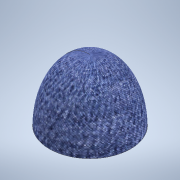
# Autodesk Inventor part: Egg Capsule Top
Saved by Autodesk Inventor 2022 (Build 260153000, 153)
## iProperties
Created: 2022-02-15
Part Number: Egg Capsule Top
Material: Generic
Document SubType Name: Modeling
Designer: Nathan Griffith
Density: 1 g/cm^3
Appearance: Denim - Blue
Author: Nathan Griffith
Autodesk Inventor part; units mm, degrees
ref_plane "YZ Plane" through (0, 0, 0) normal (1, 0, 0) x (0, 1, 0)
ref_plane "XZ Plane" through (0, 0, 0) normal (0, 1, 0) x (-1, 0, 0)
ref_plane "XY Plane" through (0, 0, 0) normal (0, 0, 1) x (1, 0, 0)
sketch "Sketch1" plane through (0, 0, 0) normal (0, 0, 1) x (1, 0, 0)
  line L0 (18.415, -31.115) -> (-18.415, -31.115)
  line L1 (-18.415, -31.115) -> (-18.415, 31.115)
  line L2 (-18.415, 31.115) -> (0, 31.115)
  line L3 (18.415, -31.115) -> (-18.415, 31.115) construction
  line L4 (-18.415, -31.115) -> (18.415, 31.115) construction
  ellipse E0 centre (0, 0) end of major axis (0, 31.115) minor radius 18.415 (0, 31.115) -> (0, -31.115) ccw
  line L5 (0, 31.115) -> (0, -31.115)
  line L6 (-18.415, 0) -> (0, 0)
  line L7 (-18.415, 31.115) -> (18.415, 31.115) construction
  dimension "d0" = 36.83
  dimension "d1" = 62.23
  constraints: 16 end point, 4 midpoint, 3 horizontal, 1 coincident, 1 parallel, 1 perpendicular, 1 vertical, 5 other
  measures "d0" distance of L1.end L4.end
  measures "d1" distance of L0.end L1.end
revolve "Revolution1" add sketch "Sketch1" angle 360 about axis through (0, 31.115, 0) along (0, -1, 0) picked at (-3.6353, 18.7288) contours E0 L5 L6
shell "Shell1" thickness 6.35 outward yes removed faces 1 at (-4.5946, 0, -1.6348)
sketch "Sketch12" plane through (0, 0, 0) normal (0, -1, 0) x (1, 0, 0)
  circle A0 centre (0, 0) radius 18.415 projected
  point P0 (0, 0)
  point P1 (-18.415, 0)
  constraints: 1 horizontal alignment
body "Solid1"
